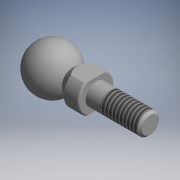
# Autodesk Inventor part: RBID6shank
Saved by Autodesk Inventor 2017.3 (Build 213256000, 256)
## iProperties
Part Number: RBID6shank
Material: Generic
Catalog Web Link: www.cadenas.de
Description: RBID, RBIDL-shank-Rod End Bearings - Link Ball Type with Thread - Link Ball Straight Type
Vendor: MISUMI
Document SubType Name: Modeling
Designer: partserver
Manufacturer: MISUMI
Mass: 1.89372 g
Surface Area: 10.203 cm^2
Volume: 1.89372 cm^3
Density: 1 g/cm^3
Appearance: PSOLRGB-192-192-192
Category: PARTsolutions
Company: MISUMI
Title: RBID6shank
Author: Cadenas PARTsolutions
Comments: Rod End Bearings - Link Ball Type with Thread - Link Ball Straight Type
PSOL_IDENT_0: {$CADENAS_DATA\23d-libs\misumi\metric\34_cylinders\rbid_shank.prj},177 {VTYP=3D},{NB=RBID6shank},{LI
PSOL_IDENT_1: NA=RBID6shank},{NN=RBID, RBIDL-shank},{DATE=30.06.2021 13:14:17},{GEOMDATE=04.07.2011 00:00:00},{VER
PSOL_IDENT_2: SION=},{LINEID=20},{WBVAR=TRS,MP},{WBNUMERIC=}  {NB=RBID6shank},{LINA=RBID6shank},{KT=DUMMY},{PN=RBI
PSOL_IDENT_3: D6},{TYPE=RBID},{TRS=1},{TRS1='1', 'Right-Hand Thread', '2', 'Left-Hand Thread'},{MATH=High Strength
PSOL_IDENT_4: Zinc Alloy},{MATS=1035 Steel},{HARDS=20~28HRC},{MATB=NBR Type Special Synthetic Rubber},{HARD=Spher
PSOL_IDENT_5: e 650HV~},{M=6},{D=10.0},{D1=13},{D2=20},{L=55.2},{L1=28},{L2=15},{MP=1},{MPA='1','M6x1.0'},{L3=5.0}
PSOL_IDENT_6: ,{W=11},{DD=6},{DDTOL=0/-0.030},{LL=27.2},{LL1=12.2},{LL2=11},{W1=8},{D3=10},{D4=20},{BD=12.700},{AS
PSOL_IDENT_7: F=25},{PK=3730},{SLCT=7450},{SLCC=14900},{MASS=40},{NDM=6},{P=1},{KDM=4.917},{PPATH=rbid_templ.prj},
PSOL_IDENT_8: {RCS=0.03 or Less},{ACS=0.1 or Less}
NB: RBID6shank
NN: RBID, RBIDL-shank
NT: Rod End Bearings - Link Ball Type with Thread - Link Ball Straight Type
NBSYN: $PN.shank
LINA: RBID6shank
CATALOG: Misumi
PN: RBID6
TRS: Right-Hand Thread
MATH: High Strength Zinc Alloy
MATS: 1035 Steel
HARDS: 20~28HRC
MATB: NBR Type Special Synthetic Rubber
HARD: Sphere 650HV~
M: 6
D: 10
D1: 13
D2: 20
L1: 28
L2: 15
MP: M6x1.0
L3: 5
W: 11
DD: 6
DDTOL: 0/-0.030
LL: 27.2
LL1: 12.2
LL2: 11
W1: 8
D3: 10
D4: 20
BD: 12.7
ASF: 25
PK: 3730
SLCT: 7450
SLCC: 14900
PPATH: rbid_templ.prj
RCS: 0.03 or Less
ACS: 0.1 or Less
SUPPLIER: MISUMI
ARTICLENO: RBID6shank
BOMINFO: RBID6shank
CREATOR: CADENAS GmbH
Autodesk Inventor part; units mm, degrees
sketch "Sketch_1" plane through (0, 0, 0) normal (0, 0, 1) x (1, 0, 0)
  line L0 (6.35, 0) -> (-27.2, 0)
  line L1 (-27.2, 0) -> (-27.2, 2.3865)
  line L2 (-27.2, 2.3865) -> (-26.5865, 3)
  line L3 (-26.5865, 3) -> (-12.2, 3)
  line L4 (-12.2, 3) -> (-12.2, 4.5)
  arc A0 (-11.7, 5) -> (-12.2, 4.5) centre (-11.7, 4.5) ccw
  line L5 (-11.7, 5) -> (-8.1333, 5)
  line L6 (-8.1333, 5) -> (-5.5967, 3)
  arc A1 (6.35, 0) -> (-5.5967, 3) centre (0, 0) ccw
  line L7 (6.35, 0) -> (-27.2, 0)
  constraints: 16 end point, 4 point on circle, 2 centre point
revolve "Revolution1" add sketch "Sketch_1" angle 360 about axis through (6.35, 0, 0) along (1, 0, 0)
thread "Thread1" size "M6x1" class "6g" standard "ISO Metric profile" length 10.3865
sketch "Sketch_2" plane through (-12.2, 0, 0) normal (1, 0, 0) x (0, 0, -1)
  line L0 (-8, 20) -> (-8, -20)
  line L1 (-8, -20) -> (8, -20)
  line L2 (8, -20) -> (8, 20)
  line L3 (8, 20) -> (-8, 20)
  line L4 (-4, 10) -> (-4, -10)
  line L5 (-4, -10) -> (4, -10)
  line L6 (4, -10) -> (4, 10)
  line L7 (4, 10) -> (-4, 10)
  constraints: 16 end point
extrude "Extrusion1" cut sketch "Sketch_2" along normal blind 6.1
ref_plane "shank_XY" through (0, 0, 0) normal (0, 0, 1) x (1, 0, 0)
ref_plane "shank_YZ" through (0, 0, 0) normal (1, 0, 0) x (0, 1, 0)
ref_plane "shank_ZX" through (0, 0, 0) normal (0, 1, 0) x (0, 0, 1)
body "Solid1"
